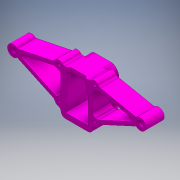
# Autodesk Inventor part: 04-08-Опора
Saved by Autodesk Inventor 2018 (Build 220112000, 112)
## iProperties
Part Number: 04-08-Опора
Material: Типовые
Document SubType Name: Modeling
Designer: sbnnl
Density: 1 g/cm^3
Appearance: Пурпурный
Author: sbnnl
Autodesk Inventor part; units mm, degrees
ref_plane "YZ Plane" through (0, 0, 0) normal (1, 0, 0) x (0, 1, 0)
ref_plane "XZ Plane" through (0, 0, 0) normal (0, 1, 0) x (-1, 0, 0)
ref_plane "XY Plane" through (0, 0, 0) normal (0, 0, 1) x (1, 0, 0)
sketch "Эскиз1" plane through (0, 0, 0) normal (0, 1, 0) x (-1, 0, 0)
  circle A0 centre (0, 0) radius 4
  line L0 (65, -38.5412) -> (65, 33.7453) construction
  circle A1 centre (65, -30) radius 2.15
  line L1 (0, 0) -> (21.7442, 0) construction
  line L2 (56.6462, -28.8978) -> (5.8522, -5.4545)
  line L3 (58.7415, -24.358) -> (13.7048, -3.5718)
  line L4 (65, -30) -> (0, 0) construction
  circle A2 centre (65, 15) radius 2.15
  arc A3 (61.5196, 10.1126) -> (63.7874, 9.1238) centre (65, 15) ccw
  line L5 (56.6155, 15.8369) -> (5.8522, 5.4545)
  line L6 (57.6174, 10.9383) -> (14.3608, 2.0912)
  arc A4 (5.8522, 5.4545) -> (5.8522, -5.4545) centre (0, 0) ccw
  arc A5 (14.3608, 2.0912) -> (13.7048, -3.5718) centre (14.9619, -0.848) ccw
  line L7 (65, 15) -> (2.1654, 2.1486) construction
  line L8 (65, 15) -> (171.4983, 15) construction
  line L9 (90, 25.4043) -> (90, -38.5412) construction
  arc A6 (69.3891, 19.0909) -> (59.8802, 18.1285) centre (65, 15) ccw
  arc A7 (63.7874, -24.1238) -> (62.7292, -24.4463) centre (65, -30) ccw
  circle A8 centre (180, 0) radius 4
  line L10 (115, -38.5412) -> (115, 33.7453) construction
  circle A9 centre (115, -30) radius 2.15
  line L11 (123.3538, -28.8978) -> (174.1478, -5.4545)
  line L12 (121.2585, -24.358) -> (166.2952, -3.5718)
  line L13 (122.3826, 10.9383) -> (165.6392, 2.0912)
  line L14 (123.3845, 15.8369) -> (174.1478, 5.4545)
  arc A10 (116.2126, 9.1238) -> (118.4804, 10.1126) centre (115, 15) ccw
  circle A11 centre (115, 15) radius 2.15
  arc A12 (174.1478, -5.4545) -> (174.1478, 5.4545) centre (180, 0) ccw
  arc A13 (166.2952, -3.5718) -> (165.6392, 2.0912) centre (165.0381, -0.848) ccw
  arc A14 (120.1198, 18.1285) -> (110.6109, 19.0909) centre (115, 15) ccw
  arc A15 (117.2708, -24.4463) -> (116.2126, -24.1238) centre (115, -30) ccw
  line L15 (0, 0) -> (180, 0)
  line L16 (106.9533, 17.5) -> (73.0467, 17.5)
  line L17 (90, 11.5) -> (90, -38.76)
  line L18 (67.7769, -19.227) -> (67.7769, 4.227)
  line L19 (112.2231, -19.227) -> (112.2231, 4.227)
  line L20 (106.2231, -46.1696) -> (73.7769, -46.1696)
  arc A16 (116.2126, -35.8762) -> (120.6995, -31.8751) centre (115, -30) ccw
  arc A17 (59.3005, -31.8751) -> (63.7874, -35.8762) centre (65, -30) ccw
  line L21 (90, -38.76) -> (73.8, -38.76)
  line L22 (90, -38.76) -> (106.2, -38.76)
  line L23 (77.8, 11.7) -> (102.2, 11.7)
  line L24 (73.8, -38.76) -> (73.8, -0.76)
  line L25 (76.8, 10.7) -> (76.8, 2.24)
  line L26 (73.8, -0.76) -> (73.8, -0.76)
  arc A18 (73.8, -0.76) -> (76.8, 2.24) centre (73.8, 2.24) ccw
  line L27 (103.2, 10.7) -> (103.2, 2.24)
  line L28 (106.2, -0.76) -> (106.2, -0.76)
  line L29 (106.2, -0.76) -> (106.2, -38.76)
  arc A19 (103.2, 2.24) -> (106.2, -0.76) centre (106.2, 2.24) ccw
  arc A20 (67.7769, 4.227) -> (63.7874, 9.1238) centre (62.7769, 4.227) ccw
  arc A21 (69.3891, 19.0909) -> (73.0467, 17.5) centre (73.0467, 22.5) ccw
  arc A22 (56.6155, 15.8369) -> (59.8802, 18.1285) centre (55.6136, 20.7355) ccw
  arc A23 (61.5196, 10.1126) -> (57.6174, 10.9383) centre (58.6193, 6.0397) ccw
  arc A24 (58.7415, -24.358) -> (62.7292, -24.4463) centre (60.8368, -19.8183) ccw
  arc A25 (63.7874, -24.1238) -> (67.7769, -19.227) centre (62.7769, -19.227) ccw
  arc A26 (59.3005, -31.8751) -> (56.6462, -28.8978) centre (54.551, -33.4376) ccw
  arc A27 (123.3538, -28.8978) -> (120.6995, -31.8751) centre (125.449, -33.4376) ccw
  arc A28 (117.2708, -24.4463) -> (121.2585, -24.358) centre (119.1632, -19.8183) ccw
  arc A29 (112.2231, -19.227) -> (116.2126, -24.1238) centre (117.2231, -19.227) ccw
  arc A30 (116.2126, 9.1238) -> (112.2231, 4.227) centre (117.2231, 4.227) ccw
  arc A31 (122.3826, 10.9383) -> (118.4804, 10.1126) centre (121.3807, 6.0397) ccw
  arc A32 (120.1198, 18.1285) -> (123.3845, 15.8369) centre (124.3864, 20.7355) ccw
  arc A33 (106.9533, 17.5) -> (110.6109, 19.0909) centre (106.9533, 22.5) ccw
  arc A34 (77.8, 11.7) -> (76.8, 10.7) centre (77.8, 10.7) ccw
  arc A35 (103.2, 10.7) -> (102.2, 11.7) centre (102.2, 10.7) ccw
  arc A36 (116.2126, -35.8762) -> (112.2231, -40.1696) centre (116.7196, -40.3475) ccw
  arc A37 (67.7769, -40.1696) -> (63.7874, -35.8762) centre (63.2804, -40.3475) ccw
  arc A38 (106.2231, -46.1696) -> (112.2231, -40.1696) centre (106.2231, -40.1696) ccw
  arc A39 (67.7769, -40.1696) -> (73.7769, -46.1696) centre (73.7769, -40.1696) ccw
  point P0 (7.4216, -0.6719)
  point P1 (60.1572, 11.4578)
  point P2 (7.4216, 0.6719)
  point P3 (59.1553, 16.3564)
  point P4 (70.4544, 17.5)
  point P5 (90, 17.5)
  point P6 (121, -29.9842)
  point P7 (119.8428, 11.4578)
  point P8 (120.8447, 16.3564)
  point P9 (109.5456, 17.5)
  point P10 (77.75, -1.96)
  point P11 (106, -46.1696)
  point P12 (112.2231, 9.6813)
  point P13 (67.7769, 9.6813)
  point P14 (59, -29.9842)
  point P15 (67.7769, -35.3187)
  point P16 (67.7769, -46.1696)
  point P17 (112.2231, -35.3187)
  point P18 (112.2231, -46.1696)
  point P19 (76.8, 11.7)
  point P20 (103.2, 11.7)
  dimension "d0" = 8
  dimension "d10" = 65
  dimension "d11" = 4.3
  dimension "d16" = 5
  dimension "d18" = 8
  dimension "d19" = 3
  dimension "d27" = 15
  dimension "d28" = 5
  dimension "d29" = 90
  dimension "d74" = 50
  dimension "d145" = 16.2
  dimension "d146" = 16.2
  dimension "d148" = 38
  dimension "d149" = 3
  dimension "d150" = 3
  dimension "d154" = 5
  dimension "d155" = 1
  dimension "d161" = 4.5
  dimension "d162" = 4.5
  dimension "d163" = 6
  dimension "d164" = 6
  constraints: 82 point on circle, 60 end point, 40 centre point, 38 tangent, 23 point on line, 19 symmetric about line, 15 equal radius, 9 coincident, 6 horizontal, 5 perpendicular, 4 parallel, 3 vertical, 10 other
  measures "d0" diameter of A0
  measures "d10" distance from line of L0 point (0, 0)
  measures "d11" diameter of A1
  measures "d16" distance between parallel lines of L3 L2
  measures "d18" radius of A4
  measures "d19" radius of A5
  measures "d27" vertical distance of A3.centre point (0, 0)
  measures "d28" distance between parallel lines of L5 L6
  measures "d29" distance from line of L9 point (0, 0)
  measures "d74" distance between parallel lines of L0 L10
  measures "d145" distance of L17.end L21.end
  measures "d146" distance of L17.end L22.end
  measures "d148" distance of L21.end L24.end
  measures "d149" radius of A18
  measures "d150" radius of A19
  measures "d154" radius of A20
  measures "d155" radius of A34
  measures "d161" radius of A36
  measures "d162" radius of A37
  measures "d163" radius of A38
  measures "d164" radius of A39
extrude "Выдавливание1" add sketch "Эскиз1" along normal blind 26
sketch "Эскиз21" plane through (0, 26, 0) normal (0, 1, 0) x (1, 0, 0)
  line L0 (-106.2, 0.76) -> (-106.2, 38.76) projected
  line L1 (-73.8, 38.76) -> (-106.2, 38.76) projected
  line L2 (-106.2, 38.76) -> (-73.8, 38.76)
  line L3 (-73.8, 38.76) -> (-73.8, 0.76) projected
  line L4 (-73.8, 38.76) -> (-73.8, 0.76)
  line L5 (-106.2, 38.76) -> (-106.2, 0.76)
  arc A0 (-103.2, -2.24) -> (-106.2, 0.76) centre (-106.2, -2.24) ccw projected
  arc A1 (-103.2, -2.24) -> (-106.2, 0.76) centre (-106.2, -2.24) ccw
  arc A2 (-73.8, 0.76) -> (-76.8, -2.24) centre (-73.8, -2.24) ccw projected
  arc A3 (-76.8, -2.24) -> (-76.8, -2.24) centre (-73.8, -2.24) ccw
  arc A4 (-77.8, -11.7) -> (-76.8, -10.7) centre (-77.8, -10.7) ccw projected
  arc A5 (-103.2, -10.7) -> (-102.2, -11.7) centre (-102.2, -10.7) ccw projected
  line L6 (-103.2, -2.24) -> (-103.2, -10.7)
  line L7 (-77.8, -11.7) -> (-102.2, -11.7) projected
  line L8 (-102.2, -11.7) -> (-77.8, -11.7)
  line L9 (-76.8, -10.7) -> (-76.8, -2.24) projected
  line L10 (-76.8, -2.24) -> (-76.8, -10.7)
  line L11 (-73.7769, 46.1696) -> (-106.2231, 46.1696) projected
  line L12 (-106.2231, 46.1696) -> (-73.7769, 46.1696)
  circle A6 centre (-65, 30) radius 2.15 projected
  arc A7 (-68.8513, 34.6008) -> (-68.8513, 25.3992) centre (-65, 30) ccw
  circle A8 centre (-115, 30) radius 2.15 projected
  line L13 (-106.9533, -17.5) -> (-73.0467, -17.5) projected
  line L14 (-67.7769, -4.227) -> (-67.7769, 19.227) projected
  arc A9 (-75.5794, -16.9347) -> (-67.7769, -4.227) centre (-82.2776, -4.0728) ccw
  arc A10 (-112.2231, -4.227) -> (-104.4207, -16.9346) centre (-97.7219, -4.0725) ccw
  arc A11 (-104.4207, -16.9346) -> (-102.1111, -17.5) centre (-102.1111, -12.5) ccw
  arc A12 (-77.8889, -17.5) -> (-75.5794, -16.9347) centre (-77.8889, -12.5) ccw
  line L15 (-67.7769, -4.227) -> (-67.7769, 23.0988)
  line L16 (-67.7769, 40.1696) -> (-67.7769, 36.9012)
  arc A13 (-106.2, 46.1696) -> (-106.2231, 46.1696) centre (-106.2231, 40.1696) ccw
  arc A14 (-67.7769, 23.0988) -> (-68.8513, 25.3992) centre (-70.7769, 23.0988) ccw
  arc A15 (-68.8513, 34.6008) -> (-67.7769, 36.9012) centre (-70.7769, 36.9012) ccw
  line L17 (-102.1111, -17.5) -> (-77.8889, -17.5)
  line L18 (-73.0467, -17.5) -> (-106.9533, -17.5) projected
  arc A16 (-111.1487, 25.3992) -> (-111.1487, 34.6008) centre (-115, 30) ccw
  arc A17 (-106.2231, 46.1696) -> (-112.2231, 40.1696) centre (-106.2231, 40.1696) ccw projected
  arc A18 (-106.2, 46.1696) -> (-112.2231, 40.1696) centre (-106.2231, 40.1696) ccw
  line L19 (-112.2231, 40.1696) -> (-112.2231, 36.9012)
  line L20 (-112.2231, -4.227) -> (-112.2231, 23.0988)
  arc A19 (-112.2231, 36.9012) -> (-111.1487, 34.6008) centre (-109.2231, 36.9012) ccw
  arc A20 (-111.1487, 25.3992) -> (-112.2231, 23.0988) centre (-109.2231, 23.0988) ccw
  arc A21 (-67.7769, 40.1696) -> (-73.7769, 46.1696) centre (-73.7769, 40.1696) ccw
  point P0 (0, 0)
  point P1 (-76.8, -17.5)
  point P2 (-103.2, -17.5)
  point P3 (-67.7769, 24.6813)
  point P4 (-67.7769, 35.3187)
  point P5 (-112.2231, 35.3187)
  point P6 (-112.2231, 24.6813)
  dimension "d158" = 14.5015
  dimension "d159" = 14.502
  dimension "d160" = 5
  dimension "d167" = 3
  constraints: 40 point on circle, 24 end point, 15 centre point, 12 tangent, 8 point on line, 5 collinear, 3 equal radius, 3 vertical, 2 coincident, 1 horizontal
  measures "d158" radius of A9
  measures "d159" radius of A10
  measures "d160" radius of A11
  measures "d167" radius of A19
extrude "Выдавливание2" add sketch "Эскиз21" along normal blind 8.75 contours A3 A2 | A21 L16 A15 A7 A14 L15 L14 A9 A12 L13 A11 A10 L20 A20 A16 A19 L19 A17 L11
sketch "Эскиз23" plane through (0, 34.75, 0) normal (0, 1, 0) x (1, 0, 0)
  arc A0 (-106.2231, 46.1696) -> (-112.2231, 40.1696) centre (-106.2231, 40.1696) ccw projected
  arc A1 (-67.7769, 40.1696) -> (-73.7769, 46.1696) centre (-73.7769, 40.1696) ccw projected
  arc A2 (-68.8513, 34.6008) -> (-67.7769, 36.9012) centre (-70.7769, 36.9012) ccw projected
  arc A3 (-67.7769, 23.0988) -> (-68.8513, 25.3992) centre (-70.7769, 23.0988) ccw projected
  arc A4 (-68.8513, 34.6008) -> (-68.8513, 25.3992) centre (-65, 30) ccw projected
  arc A5 (-68.8513, 34.6008) -> (-68.8513, 25.3992) centre (-65, 30) ccw
  arc A6 (-112.2231, 36.9012) -> (-111.1487, 34.6008) centre (-109.2231, 36.9012) ccw projected
  arc A7 (-111.1487, 25.3992) -> (-111.1487, 34.6008) centre (-115, 30) ccw projected
  arc A8 (-111.1487, 25.3992) -> (-112.2231, 23.0988) centre (-109.2231, 23.0988) ccw projected
  arc A9 (-112.2231, -4.227) -> (-104.4207, -16.9346) centre (-97.7219, -4.0725) ccw projected
  arc A10 (-104.4207, -16.9346) -> (-102.1111, -17.5) centre (-102.1111, -12.5) ccw projected
  arc A11 (-75.5794, -16.9347) -> (-67.7769, -4.227) centre (-82.2776, -4.0728) ccw projected
  arc A12 (-77.8889, -17.5) -> (-75.5794, -16.9347) centre (-77.8889, -12.5) ccw projected
  arc A13 (-77.8889, -17.5) -> (-75.5794, -16.9347) centre (-77.8889, -12.5) ccw
  line L0 (-102.1111, -17.5) -> (-77.8889, -17.5)
  line L1 (-106.2231, 46.1696) -> (-73.7769, 46.1696) projected
  line L2 (-106.2231, 46.1696) -> (-73.7769, 46.1696)
  line L3 (-112.2231, 36.9012) -> (-112.2231, 40.1696) projected
  line L4 (-112.2231, 36.9012) -> (-112.2231, 40.1696)
  line L5 (-67.7769, 36.9012) -> (-67.7769, 40.1696)
  line L6 (-112.2231, 23.0988) -> (-112.2231, -4.227) projected
  line L7 (-112.2231, -4.227) -> (-112.2231, 23.0988)
  line L8 (-67.7769, 19.227) -> (-67.7769, -4.227) projected
  line L9 (-67.7769, -4.227) -> (-67.7769, 23.0988)
  line L10 (-102.2, -11.7) -> (-77.8, -11.7) projected
  line L11 (-73.8, 38.76) -> (-106.2, 38.76) projected
  line L12 (-103.5, 6.57) -> (-103.5, 38.57)
  line L13 (-76.5, 6.57) -> (-76.5, 34.5312)
  circle A14 centre (-103.5, 6.57) radius 1.25
  circle A15 centre (-76.5, 6.57) radius 1.25
  circle A16 centre (-103.5, 14.57) radius 1.25
  circle A17 centre (-103.5, 22.57) radius 1.25
  circle A18 centre (-103.5, 30.57) radius 1.25
  circle A19 centre (-76.5, 30.57) radius 1.25
  circle A20 centre (-76.5, 22.57) radius 1.25
  circle A21 centre (-76.5, 14.57) radius 1.25
  arc A22 (-100.2, 5.1313) -> (-79.8, 5.1313) centre (-90, -0.18) ccw
  line L14 (-100.2, 32.14) -> (-79.8, 32.14)
  line L15 (-100.2, 32.14) -> (-100.2, 5.1313)
  line L16 (-79.8, 32.14) -> (-79.8, 5.1313)
  line L17 (-90, -0.18) -> (-90, 32.14)
  arc A23 (-103.2, -2.24) -> (-106.2, 0.76) centre (-106.2, -2.24) ccw projected
  circle A24 centre (-82, 35.82) radius 1.25
  circle A25 centre (-98, 35.82) radius 1.25
  point P0 (0, 0)
  dimension "d179" = 2.5
  dimension "d180" = 2.5
  dimension "d181" = 2.5
  dimension "d182" = 2.5
  dimension "d183" = 2.5
  dimension "d184" = 8
  dimension "d185" = 8
  dimension "d186" = 8
  dimension "d187" = 2.5
  dimension "d188" = 2.5
  dimension "d189" = 2.5
  dimension "d192" = 23
  dimension "d195" = 20.4
  dimension "d200" = 2.5
  dimension "d201" = 2.5
  constraints: 24 end point, 13 centre point, 7 point on circle, 5 point on line, 4 collinear, 4 vertical, 2 coincident, 2 midpoint, 1 parallel, 1 tangent
  measures "d179" diameter of A14
  measures "d180" diameter of A15
  measures "d181" diameter of A16
  measures "d182" diameter of A17
  measures "d183" diameter of A18
  measures "d184" distance of A16.centre A14.centre
  measures "d185" distance of A17.centre A16.centre
  measures "d186" distance of A18.centre A17.centre
  measures "d187" diameter of A19
  measures "d188" diameter of A20
  measures "d189" diameter of A21
  measures "d192" diameter of A22
  measures "d195" distance of L14.start L14.end
  measures "d200" diameter of A24
  measures "d201" diameter of A25
extrude "Выдавливание23" add sketch "Эскиз23" along normal blind 2.9
sketch "Эскиз24" plane through (-106.9533, 0, 17.5) normal (0, 0, 1) x (1, 0, 0)
  line L0 (3.7533, 0) -> (3.7533, 34.75) projected
  line L1 (3.7533, 0) -> (3.7533, 0)
  line L2 (6.7533, 3) -> (26.1533, 3)
  line L3 (29.1533, 0) -> (29.1533, 34.75) projected
  line L4 (29.1533, 0) -> (29.1533, 0)
  line L5 (29.1533, 0) -> (3.7533, 0)
  line L6 (33.9065, 0) -> (0, 0) projected
  arc A0 (6.7533, 3) -> (3.7533, 0) centre (6.7533, 0) ccw
  arc A1 (29.1533, 0) -> (26.1533, 3) centre (26.1533, 0) ccw
  point P0 (106.9533, 0)
  point P1 (3.7533, 3)
  point P2 (29.1533, 3)
  dimension "d205" = 3
  dimension "d206" = 3
  constraints: 8 end point, 6 point on line, 4 point on circle, 4 tangent, 2 centre point, 1 collinear, 1 equal radius, 1 perpendicular, 1 vertical
  measures "d205" distance of L0.start point (3.753, 3)
  measures "d206" radius of A0
extrude "Выдавливание24" cut sketch "Эскиз24" against normal blind 6
sketch "Эскиз25" plane through (0, 26, 0) normal (0, 1, 0) x (1, 0, 0)
  circle A0 centre (0, 0) radius 4 projected
  circle A1 centre (0, 0) radius 5
  circle A2 centre (-180, 0) radius 4 projected
  circle A3 centre (-180, 0) radius 5
  dimension "d209" = 10
  dimension "d210" = 10
  constraints: 2 centre point, 2 coincident
  measures "d209" diameter of A1
  measures "d210" diameter of A3
extrude "Выдавливание25" cut sketch "Эскиз25" against normal blind 0.7
sketch "Эскиз26" plane through (0, 0, 0) normal (0, -1, 0) x (1, 0, 0)
  circle A0 centre (0, 0) radius 4 projected
  circle A1 centre (0, 0) radius 5
  circle A2 centre (-180, 0) radius 4 projected
  circle A3 centre (-180, 0) radius 5
  dimension "d213" = 10
  dimension "d214" = 10
  constraints: 2 centre point, 2 coincident
  measures "d213" diameter of A1
  measures "d214" diameter of A3
extrude "Выдавливание26" cut sketch "Эскиз26" against normal blind 0.7
sketch "Эскиз27" plane through (0, 0, 0) normal (0, -1, 0) x (1, 0, 0)
  line L0 (-106.2, -38.76) -> (-106.2, -0.76) projected
  line L1 (-106.2, -38.76) -> (-106.2, -0.76)
  line L2 (-106.2, -38.76) -> (-105.5, -38.76)
  line L3 (-106.2, -38.76) -> (-73.8, -38.76) projected
  line L4 (-105.5, -38.76) -> (-105.5, -0.6772)
  arc A0 (-106.2, -0.76) -> (-103.2, 2.24) centre (-106.2, 2.24) ccw projected
  arc A1 (-106.2, -0.76) -> (-105.5, -0.6772) centre (-106.2, 2.24) ccw
  line L5 (-73.8, -0.76) -> (-73.8, -38.76) projected
  line L6 (-73.8, -38.76) -> (-74.5, -38.76)
  line L7 (-74.5, -38.76) -> (-74.5, -0.6772)
  arc A2 (-76.8, 2.24) -> (-73.8, -0.76) centre (-73.8, 2.24) ccw projected
  arc A3 (-74.5, -0.6772) -> (-73.8, -0.76) centre (-73.8, 2.24) ccw
  line L8 (-73.8, -0.76) -> (-73.8, -38.76)
  point P0 (0, 0)
  dimension "d217" = 0.7
  dimension "d218" = 0.7
  constraints: 12 end point, 6 point on circle, 2 centre point, 2 collinear, 2 concentric, 2 point on line, 1 perpendicular, 1 vertical
  measures "d217" distance of L0.start L2.end
  measures "d218" distance of L3.end L6.end
extrude "Выдавливание27" add sketch "Эскиз27" against normal blind 3
chamfer "Фаска6" distance 0.7 angle 45 4 edges at (-105.5, 3, -19.7186) (-74.5, 3, -19.7186) (-105.5, 0, -19.7186) (-74.5, 0, -19.7186)
